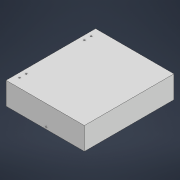
# Autodesk Inventor part: Ebene3_hinten
Saved by Autodesk Inventor 2021 (Build 250183000, 183)
## iProperties
Created: 2021-02-07
Part Number: Ebene3_hinten
Material: Generisch
Document SubType Name: Modeling
Designer: laure
Density: 1 g/cm^3
Appearance: Vorgabe
Author: laure
## iProperties of the stored document _3D-Druck.ipt
Created: 2021-03-02
Part Number: _3D-Druck
Material: Generisch
Document SubType Name: Modeling
Designer: Ctroi
Density: 1 g/cm^3
Appearance: Vorgabe
Author: Ctroi
Autodesk Inventor part; units mm, degrees
ref_plane "YZ Plane" through (0, 0, 0) normal (1, 0, 0) x (0, 1, 0)
ref_plane "XZ Plane" through (0, 0, 0) normal (0, 1, 0) x (-1, 0, 0)
ref_plane "XY Plane" through (0, 0, 0) normal (0, 0, 1) x (1, 0, 0)
sketch "Skizze1" plane through (0, 0, 0) normal (0, 1, 0) x (-1, 0, 0)
  line L0 (87.5, -100) -> (-87.5, -100)
  line L1 (-87.5, -100) -> (-87.5, 100)
  line L2 (-87.5, 100) -> (87.5, 100)
  line L3 (87.5, 100) -> (87.5, -100)
  line L4 (0, -140) -> (0, 140) projected
  line L5 (-122.5, 0) -> (122.5, 0) projected
  point P0 (0, 0)
  dimension "d0" = 175
  dimension "d1" = 200
  constraints: 8 end point, 2 parallel, 1 horizontal, 1 perpendicular, 2 other
  measures "d0" distance between parallel lines of L1 L3
  measures "d1" distance between parallel lines of L2 L0
extrude "Extrusion1" add sketch "Skizze1" along normal mid plane 2
sketch "Skizze2" plane through (0, -1, 0) normal (0, -1, 0) x (1, 0, 0)
  line L0 (-87.5, -100) -> (-87.5, 100) projected
  line L1 (87.5, 100) -> (87.5, -100) projected
  line L2 (-87.5, 100) -> (87.5, 100)
  line L3 (87.5, 100) -> (87.5, 98)
  line L4 (87.5, 98) -> (-87.5, 98)
  line L5 (-87.5, 98) -> (-87.5, 100)
  line L6 (87.5, -100) -> (-87.5, -100) projected
  line L7 (-87.5, -100) -> (87.5, -100)
  line L8 (87.5, -100) -> (87.5, -98)
  line L9 (87.5, -98) -> (-87.5, -98)
  line L10 (-87.5, -98) -> (-87.5, -100)
  line L11 (87.5, -98) -> (85.5, -98)
  line L12 (85.5, -98) -> (85.5, 98)
  line L13 (85.5, 98) -> (87.5, 98)
  line L14 (87.5, 98) -> (87.5, -98)
  point P0 (0, 0)
  dimension "d4" = 2
  dimension "d5" = 2
  dimension "d6" = 2
  constraints: 24 end point, 6 parallel, 3 horizontal, 3 perpendicular, 3 point on line
  measures "d4" distance of L2.end L3.end
  measures "d5" distance of L8.end L7.end
  measures "d6" distance of L12.end L13.end
extrude "Extrusion2" add sketch "Skizze2" along normal blind 48 contours L0 L9 L1 L6 | L0 L2 L1 L4 | L12 L4 L1 L9
sketch "Skizze3" plane through (0, 1, 0) normal (0, 1, 0) x (1, 0, 0)
  circle A0 centre (-77.5, -80) radius 1.6
  circle A1 centre (-77.5, -65) radius 1.6
  circle A2 centre (-77.5, 80) radius 1.6
  circle A3 centre (-77.5, 65) radius 1.6
  line L0 (-87.5, 100) -> (-87.5, -100) projected
  line L1 (-87.5, -100) -> (87.5, -100) projected
  line L2 (87.5, 100) -> (-87.5, 100) projected
  point P0 (0, 0)
  dimension "d9" = 3.2
  dimension "d10" = 3.2
  dimension "d11" = 3.2
  dimension "d12" = 3.2
  dimension "d13" = 10
  dimension "d14" = 10
  dimension "d15" = 15
  dimension "d16" = 20
  dimension "d17" = 10
  dimension "d18" = 10
  dimension "d19" = 20
  dimension "d20" = 15
  constraints: 4 centre point
  measures "d9" diameter of A0
  measures "d10" diameter of A1
  measures "d11" diameter of A2
  measures "d12" diameter of A3
  measures "d13" distance from line of L0 A0.centre
  measures "d14" distance from line of L0 A1.centre
  measures "d15" distance of A1.centre A0.centre
  measures "d16" distance from line of L1 A0.centre
  measures "d17" distance from line of L0 A3.centre
  measures "d18" distance from line of L0 A2.centre
  measures "d19" distance from line of A2.centre L2
  measures "d20" distance of A3.centre A2.centre
extrude "Extrusion3" cut sketch "Skizze3" against normal up to surface (2 mm away)
sketch "Skizze4" plane through (-87.5, 1, 100) normal (0, 0, 1) x (1, 0, 0)
  circle A0 centre (90, -45) radius 1.6
  line L0 (175, -50) -> (175, 0) projected
  line L1 (175, -50) -> (0, -50) projected
  point P0 (87.5, -1)
  dimension "d23" = 3.2
  dimension "d24" = 85
  dimension "d25" = 5
  constraints: 1 centre point
  measures "d23" diameter of A0
  measures "d24" distance from line of L0 A0.centre
  measures "d25" distance from line of A0.centre L1
extrude "Extrusion4" cut sketch "Skizze4" against normal up to surface (2 mm away)
sketch "Skizze5" plane through (87.5, 1, -100) normal (0, 0, -1) x (-1, 0, 0)
  circle A0 centre (85, -45) radius 1.6
  line L0 (175, -50) -> (0, -50) projected
  line L1 (0, -50) -> (0, 0) projected
  point P0 (87.5, -1)
  dimension "d28" = 3.2
  dimension "d29" = 5
  dimension "d30" = 85
  constraints: 1 centre point
  measures "d28" diameter of A0
  measures "d29" distance from line of L0 A0.centre
  measures "d30" distance from line of L1 A0.centre
extrude "Extrusion5" cut sketch "Skizze5" against normal up to surface (2 mm away)
